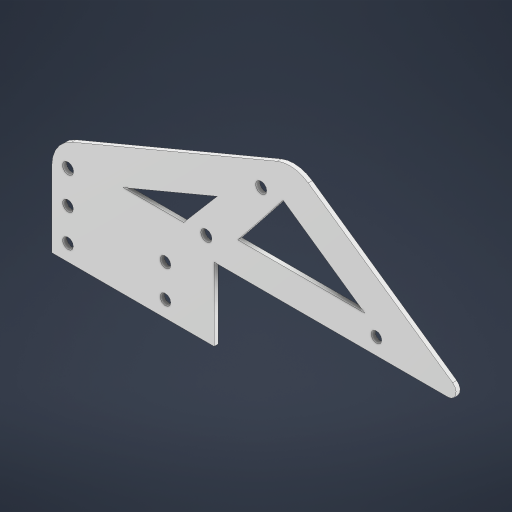
# Autodesk Inventor part: plate_right
Saved by Autodesk Inventor 2024 (Build 280153000, 153)
## iProperties
Created: 2023-11-09
Part Number: plate_right
Material: Acetal Resin, White
Document SubType Name: Modeling
Designer: avere
Density: 1.425 g/cm^3
Appearance: Smooth - White
Author: avere
Autodesk Inventor part; units mm, degrees
ref_plane "YZ Plane" through (0, 0, 0) normal (1, 0, 0) x (0, 1, 0)
ref_plane "XZ Plane" through (0, 0, 0) normal (0, 1, 0) x (-1, 0, 0)
ref_plane "XY Plane" through (0, 0, 0) normal (0, 0, 1) x (1, 0, 0)
sketch "Sketch1" plane through (0, 0, 0) normal (0, 0, 1) x (1, 0, 0)
  circle A0 centre (0, 0) radius 2.0955
  circle A1 centre (0, 12.7) radius 2.0955
  line L0 (-6.35, -6.35) -> (-6.35, 23.3043)
  line L1 (81.7912, 68.7124) -> (1.4386, 35.0162)
  line L2 (57.15, -6.35) -> (57.15, 9.525)
  line L3 (-6.35, -6.35) -> (57.15, -6.35)
  line L4 (57.15, 22.225) -> (148.6454, 22.225)
  circle A2 centre (0, 25.4) radius 2.1844
  arc A3 (1.4386, 35.0162) -> (-6.35, 23.3043) centre (6.35, 23.3043) ccw
  line L5 (57.15, -6.35) -> (57.15, 22.225)
  line L6 (45.2425, 29.699) -> (58.3779, 45.1224)
  line L7 (66.4245, 34.39) -> (84.1386, 56.6755)
  line L8 (84.1386, 56.6755) -> (116.0822, 34.39)
  line L9 (93.9691, 67.4163) -> (150.462, 28.0039)
  line L10 (116.0822, 34.39) -> (66.4245, 34.39)
  line L11 (45.2425, 29.699) -> (21.5989, 29.699)
  line L12 (21.5989, 29.699) -> (58.3779, 45.1224)
  circle A4 centre (75.5451, 56.6755) radius 2.1844
  circle A5 centre (54.1023, 29.699) radius 2.1844
  circle A6 centre (38.1, 0) radius 2.0955
  circle A7 centre (38.1, 12.7) radius 2.0955
  circle A8 centre (120.65, 28.575) radius 2.0955
  arc A9 (148.6454, 22.225) -> (150.462, 28.0039) centre (148.6454, 25.4) ccw
  arc A10 (93.9691, 67.4163) -> (81.7912, 68.7124) centre (86.7026, 57.0006) ccw
  point P0 (-6.35, 31.75)
  point P1 (146.05, 22.225)
  point P2 (82.55, 22.225)
  point P3 (126.3723, 44.8101)
  point P4 (100.0585, 63.168)
  point P5 (57.15, 9.525)
  dimension "d8" = 4.191
  dimension "d9" = 4.191
  dimension "d11" = 38.1
  dimension "d22" = 63.5
  dimension "d27" = 4.3688
  dimension "d28" = 12.7
  dimension "d35" = 28.575
  dimension "d98" = 4.3688
  dimension "d99" = 4.3688
  dimension "d100" = 4.191
  dimension "d101" = 4.191
  dimension "d105" = 3.175
  dimension "d106" = 12.7
  constraints: 26 end point, 11 centre point, 7 point on line, 6 point on circle, 6 tangent, 3 horizontal, 3 vertical, 1 coincident, 1 parallel, 1 perpendicular, 3 other
  measures "d8" diameter of A0
  measures "d9" diameter of A1
  measures "d11" distance of L0.start point (-6.35, 31.75)
  measures "d22" distance of L0.start L2.start
  measures "d27" diameter of A2
  measures "d28" radius of A3
  measures "d35" distance of L2.start L5.end
  measures "d98" diameter of A4
  measures "d99" diameter of A5
  measures "d100" diameter of A6
  measures "d101" diameter of A7
  measures "d105" radius of A9
  measures "d106" radius of A10
extrude "Extrusion1" add sketch "Sketch1" along normal blind 1.5875
body "Solid1"
